Wheel adapter_v1 (Autodesk Fusion 360 design; units mm, degrees)
Autodesk Fusion 360 part; units mm, degrees
sketch "Sketch1" plane through (0, 0, 0) normal (0, 0, 1) x (1, 0, 0) in component "Component"
  circle A0 centre (0, 0) radius 5.75
  circle A1 centre (0, 0) radius 3
  dimension "d1" = 11.5
  dimension "d2" = 6
  constraint coincident A0.centre A1.centre
  measures "d1" diameter of A0
  measures "d2" diameter of A1
extrude "Extrude1" add sketch "Sketch1" along normal blind 12 in component "Component"
sketch "Sketch2" plane through (0, 0, 12) normal (0, 0, 1) x (-1, 0, 0) in component "Component"
  circle A0 centre (0, 0) radius 3
  circle A1 centre (0, 0) radius 5.75
  circle A2 centre (0, 0) radius 2
  line L0 (-6, 3.4641) -> (-6, -3.4641)
  line L1 (-6, -3.4641) -> (0, -6.9282)
  line L2 (0, -6.9282) -> (6, -3.4641)
  line L3 (6, -3.4641) -> (6, 3.4641)
  line L4 (6, 3.4641) -> (0, 6.9282)
  line L5 (0, 6.9282) -> (-6, 3.4641)
  dimension "d5" = 4
  dimension "d6" = 6
  constraint coincident A0.centre A1.centre
  constraint vertical L0
  measures "d5" diameter of A2
  measures "d6" distance of A0.centre L5
extrude "Extrude2" add sketch "Sketch2" along normal blind 6 contours A0 | A1 | L0 L1 L2 L3 L4 L5 in component "Component"
component "Component" placed x (1, 0, 0) y (0, 1, 0) z (0, 0, 1) at (0, 0, 0)
